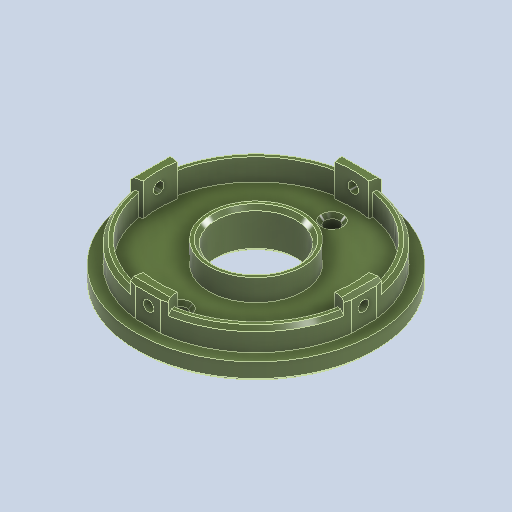
# Autodesk Inventor part: back_sleeve
Saved by Autodesk Inventor 2025 (Build 290162000, 162)
## iProperties
Created: 2026-08-15
Part Number: back_sleeve
Material: Ogólny
Document SubType Name: Modeling
Designer: zzapa
Density: 1 g/cm^3
Appearance: Ciemnooliwkowa
Author: zzapa
Autodesk Inventor part; units mm, degrees
note: some values were not read from the file. Chosen so that the rebuilt part matches the saved one: direction of "Otwór2".
ref_plane "YZ Plane" through (0, 0, 0) normal (1, 0, 0) x (0, 1, 0)
ref_plane "XZ Plane" through (0, 0, 0) normal (0, 1, 0) x (-1, 0, 0)
ref_plane "XY Plane" through (0, 0, 0) normal (0, 0, 1) x (1, 0, 0)
sketch "Szkic1" plane through (0, 0, 0) normal (0, 1, 0) x (-1, 0, 0)
  circle A0 centre (0, 0) radius 11.1
  circle A1 centre (0, 0) radius 33
  dimension "d0" = 66
  dimension "d1" = 22.2
  constraints: 2 centre point, 2 coincident
  measures "d0" diameter of A1
  measures "d1" diameter of A0
sketch "Szkic1 outline for Wyciągnięcie proste1" plane through (0, 0, 0) normal (0, 1, 0) x (-1, 0, 0)
  circle A0 centre (0, 0) radius 33
  circle A1 centre (0, 0) radius 11.1
extrude "Wyciągnięcie proste1" add sketch "Szkic1 outline for Wyciągnięcie proste1" along normal blind 5
sketch "Szkic2" plane through (0, 5, 0) normal (0, 1, 0) x (1, 0, 0)
  circle A0 centre (0, 0) radius 11.1
  circle A1 centre (0, 0) radius 13
  circle A2 centre (0, 0) radius 11.1 projected
  circle A3 centre (0, 0) radius 27.9
  circle A4 centre (0, 0) radius 29.9
  dimension "d4" = 26
  dimension "d7" = 59.8
  dimension "d8" = 2
  constraints: 4 centre point, 4 coincident, 1 concentric
  measures "d4" diameter of A1
  measures "d7" diameter of A4
  measures "d8" radial gap between concentric circles of A4 A3
sketch "Szkic2 outline for Wyciągnięcie proste2" plane through (0, 5, 0) normal (0, 1, 0) x (1, 0, 0)
  circle A0 centre (0, 0) radius 13
  circle A1 centre (0, 0) radius 11.1
  circle A2 centre (0, 0) radius 29.9
  circle A3 centre (0, 0) radius 27.9
extrude "Wyciągnięcie proste2" add sketch "Szkic2 outline for Wyciągnięcie proste2" along normal blind 6
sketch "Szkic3" plane through (0, 5, 0) normal (0, 1, 0) x (1, 0, 0)
  line L0 (46.2, 0) -> (-46.2, 0) projected
  line L1 (0, 46.2) -> (0, -46.2) projected
  point P0 (0, 0)
  point P1 (0, 21)
  point P2 (0, -21)
  dimension "d12" = 21
  constraints: 1 point on line, 1 symmetric about line
  measures "d12" distance of point (0, 21) point (0, 0)
hole "Otwór1" at (0, 5, -21) at (0, 5, 21) direction (0, -1, 0) diameter 4 end through all
sketch "Szkic4" plane through (0, 0, 0) normal (0, 0, 1) x (1, 0, 0)
  line L0 (-26.9, 5) -> (-29.9, 5)
  line L1 (-29.9, 5) -> (-29.9, 14)
  line L2 (-29.9, 14) -> (-26.9, 14)
  line L3 (-26.9, 14) -> (-26.9, 5)
  line L4 (27.9, 5) -> (-27.9, 5)
  line L5 (-29.9, 5) -> (-29.9, 11)
  line L6 (0, -4.279438) -> (0, 25.676629)
  point P0 (0, 0)
  dimension "d23" = 9
  dimension "d24" = 3
  constraints: 8 end point, 2 collinear, 2 parallel, 1 horizontal, 1 perpendicular
  measures "d23" distance between parallel lines of L2 L4
  measures "d24" distance between parallel lines of L1 L3
sketch "Szkic4 outline for Obrót1" plane through (0, 0, 0) normal (0, 0, 1) x (1, 0, 0)
  line L0 (-26.9, 14) -> (-29.9, 14)
  line L1 (-26.9, 5) -> (-26.9, 14)
  line L2 (-29.9, 5) -> (-26.9, 5)
  line L3 (-29.9, 14) -> (-29.9, 5)
revolve "Obrót1" add sketch "Szkic4 outline for Obrót1" angle 20 mid plane about axis through (0, -10, 0) along (0, 1, 0)
sketch "Szkic5" plane through (0, 14, 0) normal (0, 1, 0) x (1, 0, 0)
  arc A0 (-29.445752, 5.192081) -> (-29.445752, -5.192081) centre (0, 0) ccw
  line L0 (-29.9, 3.452535) -> (-29.7, 3.452535)
  line L1 (-29.7, 3.452535) -> (-29.7, -3.452535)
  line L2 (-29.7, -3.452535) -> (-29.9, -3.452535)
  line L3 (-29.9, -3.452535) -> (-29.9, 3.452535)
  line L4 (-46.2, 0) -> (46.2, 0)
  point P0 (0, 0)
  point P1 (-29.9, 0)
  point P2 (-29.9, 0)
  dimension "d25" = 0.2
  constraints: 8 end point, 2 midpoint, 2 parallel, 2 point on circle, 1 horizontal, 1 perpendicular, 1 point on line
  measures "d25" distance between parallel lines of L3 L1
sketch "Szkic5 outline for Wyciągnięcie proste3" plane through (0, 14, 0) normal (0, 1, 0) x (1, 0, 0)
  line L0 (-29.7, -3.452535) -> (-29.7, 3.452535)
  line L1 (-29.9, -3.452535) -> (-29.7, -3.452535)
  line L2 (-29.9, 3.452535) -> (-29.9, -3.452535)
  line L3 (-29.7, 3.452535) -> (-29.9, 3.452535)
extrude "Wyciągnięcie proste3" cut sketch "Szkic5 outline for Wyciągnięcie proste3" against normal up to surface (9 mm away)
sketch "Szkic6" plane through (-29.7, 14, -3.452535) normal (-1, 0, 0) x (0, 0, 1)
  line L0 (8.297319, -3) -> (8.644616, -3)
  line L1 (8.644616, -3) -> (-1.739545, -3)
  line L2 (-1.739545, -3) -> (-1.392249, -3)
  line L3 (-1.392249, -3) -> (8.297319, -3)
  line L4 (0, 0) -> (6.905071, 0)
  line L5 (8.123671, 0) -> (-1.218601, 0)
  line L6 (3.452535, 0) -> (3.452535, -3)
  line L7 (36.452535, -9) -> (-29.547465, -9)
  point P0 (3.452535, -14)
  point P1 (3.452535, -4.1)
  dimension "d34" = 4.9
  constraints: 2 end point, 2 midpoint, 1 point on line
  measures "d34" distance from line of L7 point (3.453, -4.1)
hole "Otwór2" at (-29.7, 9.9, 0) direction (1, 0, 0) diameter 2.9 end up to surface
pattern_circular "Szyk kołowy1" count 4 over 360 about axis through (0, -10, 0) along (0, 1, 0) of "Obrót1", "Wyciągnięcie proste3", "Otwór2"
chamfer "Faza1" distance 1 angle 45 15 edges at (33, 0, 0) (11.1, 0, 0) (-11.1, 11, 0) (0, 5, 19) (0, 5, -23) (0, 0, -23) (0, 0, 19) (21.1425, 11, -21.1425) (29.7, 14, 0) (21.1425, 11, 21.1425) (0, 14, 29.7) (-21.1425, 11, 21.1425) (-29.7, 14, 0) (-21.1425, 11, -21.1425) (0, 14, -29.7)
equation "\"d0\" = back_sleeve_D"
equation "\"d1\" = back_sleeve_d"
equation "\"d2\" = back_sleeve_h"
equation "\"d4\" = back_sleeve_bearing_cup_d"
equation "\"d7\" = back_sleeve_bearing_casing_out_d"
equation "\"d8\" = back_sleeve_bearing_casing_out_width"
equation "\"d5\" = back_sleeve_bearing_cup_h"
equation "\"d12\" = back_sleeve_cable_hole_pos"
equation "\"d13\" = back_sleeve_cable_hole_d"
equation "\"d15\" = insert_m2_pocket_D"
equation "\"d16\" = insert_m2_pocket_nut_h"
equation "\"d23\" = back_sleeve_casing_conn_h"
equation "\"d24\" = back_sleeve_casing_conn_a"
equation "\"d20\" = back_sleeve_casing_conn_ang"
equation "\"d25\" = back_sleeve_casing_conn_cut"
equation "\"d34\" = back_sleeve_casing_conn_insert_pos"
equation "\"d27\" = insert_m2_d"
equation "\"d9\" = back_sleeve_corner"
equation "\"insert_m2_d\" = 2.9"
equation "\"insert_m2_h\" = 7"
equation "\"insert_m2_corner\" = 0.5"
equation "\"insert_m2_pocket_d\" = 2.6"
equation "\"insert_m2_pocket_D\" = 4.5"
equation "\"insert_m2_pocket_nut_h\" = 1.5"
equation "\"stator_r_out\" = 30.15"
equation "\"stator_out_d\" = 3.2"
equation "\"stator_h\" = 45"
equation "\"stator_radial_screw_d\" = 4"
equation "\"stator_radial_screw_pos\" = 4"
equation "\"mag_size_x\" = 7"
equation "\"mag_size_y\" = 3"
equation "\"mag_corner_r\" = 0.4"
equation "\"magnet_ring_r\" = 26.95"
equation "\"magnet_ring_d\" = 3.3"
equation "\"magnet_ring_h\" = 36"
equation "\"magnet_ring_pocket_mag_size_x\" = 7.1"
equation "\"magnet_ring_pocket_mag_size_y\" = 3.1"
equation "\"magnet_ring_pocket_mag_size_z\" = 10.1"
equation "\"magnet_ring_pocket_radial_cut\" = 1.4"
equation "\"magnet_ring_insert_part_lengthen\" = 8"
equation "\"magnet_ring_insert_part_axial_flat_cut\" = 0.17"
equation "\"magnet_ring_insert_pos\" = 4"
equation "\"casing_d\" = 3"
equation "\"casing_r_in\" = 30.15"
equation "\"casing_lock_hole_r\" = 14.25"
equation "\"casing_lock_h\" = 8"
equation "\"casing_stator_fix_r\" = 23"
equation "\"casing_stator_fix_h\" = 6"
equation "\"casing_sidebar_length\" = 3"
equation "\"casing_vent_hole_length\" = 4"
equation "\"casing_vent_hole_width\" = 6"
equation "\"casing_head_insert_r\" = 19"
equation "\"casing_radial_stator_insert_pos\" = 18.1"
equation "\"casing_cart_hole_ang\" = 90deg"
equation "\"casing_cart_hole_width\" = 2.6"
equation "\"casing_cart_hole_corner\" = 1"
equation "\"casing_cart_hole_pos\" = 17"
equation "\"casing_sleeve_cut_d\" = 46"
equation "\"casing_sleeve_cut_h\" = 4"
equation "\"casing_backsleeve_insert_pos\" = 4.9"
equation "\"rotor_out_r\" = 22.5"
equation "\"rotor_coil_groove_in_r\" = 17"
equation "\"rotor_coil_groove_ang\" = 18deg"
equation "\"rotor_core_r\" = 14.97"
equation "\"rotor_coil_groove_in_correction_r\" = 18"
equation "\"rotor_plastic_h\" = 32"
equation "\"rotor_teeth_d\" = 1.5"
equation "\"rotor_plastic_insert_r\" = 37"
equation "\"shaft_d\" = 8"
equation "\"shaft_lock_1_d\" = 8.1"
equation "\"shaft_lock_1_D\" = 44"
equation "\"shaft_lock_1_h1\" = 3.5"
equation "\"shaft_lock_1_corner\" = 2"
equation "\"shaft_lock_1_rotor_insert_grove_d_in\" = 36"
equation "\"shaft_lock_1_rotor_insert_grove_width_out\" = 5.5"
equation "\"shaft_lock_1_rotor_insert_grove_width_in\" = 7.6"
equation "\"shaft_lock_1_rotor_insert_r\" = 37"
equation "\"shaft_lock_1_shaft_insert_axial_cut_out_width\" = 12"
equation "\"shaft_lock_1_shaft_insert_axial_cut_in_width\" = 5.4"
equation "\"shaft_lock_1_shaft_insert_pos\" = 2.5"
equation "\"shaft_lock_1_shaft_insert_corner\" = 2"
equation "\"shaft_lock_1_shaft_insert_corner_finish\" = 0.5"
equation "\"shaft_lock_2_d\" = 8.1"
equation "\"shaft_lock_2_D\" = 44"
equation "\"shaft_lock_2_h1\" = 3.5"
equation "\"shaft_lock_2_corner\" = 2"
equation "\"shaft_lock_2_rotor_insert_grove_d_in\" = 36"
equation "\"shaft_lock_2_rotor_insert_grove_width_out\" = 5.5"
equation "\"shaft_lock_2_rotor_insert_grove_width_in\" = 7.6"
equation "\"shaft_lock_2_rotor_insert_r\" = 37"
equation "\"shaft_lock_2_shaft_insert_axial_cut_out_width\" = 12"
equation "\"shaft_lock_2_shaft_insert_axial_cut_in_width\" = 5.4"
equation "\"shaft_lock_2_shaft_insert_pos\" = 2.5"
equation "\"shaft_lock_2_shaft_insert_corner\" = 2"
equation "\"shaft_lock_2_shaft_insert_corner_finish\" = 0.5"
equation "\"commutator_plastic_shaft_d\" = 8.1"
equation "\"commutator_plastic_h\" = 17"
equation "\"commutator_plastic_insert_cut_deepness\" = 0.5"
equation "\"commutator_plastic_insert_cut_length\" = 6"
equation "\"commutator_plastic_insert_pos\" = 3"
equation "\"commutator_plate_D\" = 22"
equation "\"commutator_plate_d\" = 1"
equation "\"commutator_plate_ang\" = 55deg"
equation "\"commutator_plate_h\" = 17"
equation "\"commutator_plate_insert_pos\" = 3"
equation "\"sleeve_in_r\" = 11.1"
equation "\"sleeve_d\" = 3"
equation "\"sleeve_h\" = 7"
equation "\"sleeve_cup_r\" = 22"
equation "\"sleeve_cup_h\" = 4.5"
equation "\"sleeve_head_insert_r\" = 19"
equation "\"sleeve_bearing_material_lock_h\" = 2"
equation "\"rotor_sleeve_in_D\" = 8.15"
equation "\"rotor_sleeve_out_D\" = 10.5"
equation "\"rotor_sleeve_h\" = 32"
equation "\"carbon_brush_batt_d\" = 4"
equation "\"carbon_brush_batt_h\" = 8"
equation "\"brush_cart_outer_holder_width\" = 5.5"
equation "\"brush_cart_outer_holder_arc_r\" = 33.15"
equation "\"brush_cart_outer_holder_arc_pos\" = 1.5"
equation "\"brush_holder_batt_width\" = 16"
equation "\"brush_holder_batt_arc_r\" = 30.15"
equation "\"brush_holder_batt_insert_flat_length\" = 6"
equation "\"brush_holder_batt_insert_flat_depth\" = 6"
equation "\"brush_holder_batt_brush_hole_d\" = 4.5"
equation "\"name_plate_D\" = 45"
equation "\"name_plate_d\" = 28"
equation "\"name_plate_insert_r\" = 19"
equation "\"back_sleeve_D\" = 66"
equation "\"back_sleeve_d\" = 22.2"
equation "\"back_sleeve_h\" = 5"
equation "\"commutator_back_plate_lock_h\" = 2"
equation "\"commutator_back_plate_lock_r\" = 23"
equation "\"commutator_plastic_back_plate_lock_r\" = 11.9"
equation "\"commutator_plastic_back_plate_lock_h\" = 1"
equation "\"commutator_plastic_back_plate_hook_in_r\" = 11.15"
equation "\"commutator_plastic_back_plate_hook_d\" = 1"
equation "\"commutator_plastic_back_plate_hook_h\" = 1"
equation "\"back_sleeve_bearing_cup_d\" = 26"
equation "\"back_sleeve_bearing_casing_out_d\" = 59.8"
equation "\"back_sleeve_bearing_casing_out_width\" = 2"
equation "\"back_sleeve_bearing_cup_h\" = 6"
equation "\"back_sleeve_cable_hole_d\" = 4"
equation "\"back_sleeve_casing_conn_h\" = 9"
equation "\"back_sleeve_casing_conn_a\" = 3"
equation "\"back_sleeve_casing_conn_ang\" = 20deg"
equation "\"back_sleeve_casing_conn_cut\" = 0.2"
equation "\"back_sleeve_corner\" = 1"
equation "\"back_sleeve_cable_hole_pos\" = 21"
equation "\"back_sleeve_casing_conn_insert_pos\" = 4.9"
